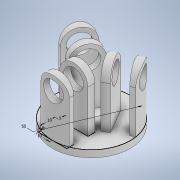
# Autodesk Inventor part: Base
Saved by Autodesk Inventor 2022 (Build 260153000, 153)
## iProperties
Created: 2022-10-13
Part Number: Base
Material: Generic
Document SubType Name: Modeling
Designer: Jasper
Density: 1 g/cm^3
Appearance: Default
Author: Jasper
Autodesk Inventor part; units mm, degrees
ref_plane "YZ Plane" through (0, 0, 0) normal (1, 0, 0) x (0, 1, 0)
ref_plane "XZ Plane" through (0, 0, 0) normal (0, 1, 0) x (-1, 0, 0)
ref_plane "XY Plane" through (0, 0, 0) normal (0, 0, 1) x (1, 0, 0)
sketch "Sketch1" plane through (0, 0, 0) normal (0, 1, 0) x (-1, 0, 0)
  circle A0 centre (0, 0) radius 27.5
  line L0 (0, 27.5) -> (10, 27.5)
  line L1 (10, 27.5) -> (10, 22.5)
  line L2 (10, 22.5) -> (0, 22.5)
  line L3 (0, 22.5) -> (0, 27.5)
  line L4 (10, 12.5) -> (0, 12.5)
  line L5 (0, 12.5) -> (0, 7.5)
  line L6 (0, 7.5) -> (10, 7.5)
  line L7 (10, 7.5) -> (10, 12.5)
  line L8 (0, 27.5) -> (-10, 27.5)
  line L9 (-10, 27.5) -> (-10, 22.5)
  line L10 (-10, 22.5) -> (0, 22.5)
  line L11 (-10, 12.5) -> (0, 12.5)
  line L12 (0, 7.5) -> (-10, 7.5)
  line L13 (-10, 7.5) -> (-10, 12.5)
  point P0 (-10, 25.6174)
  point P1 (10, 25.6174)
  dimension "d0" = 55
  dimension "d1" = 5
  dimension "d2" = 5
  dimension "d3" = 10
  dimension "d4" = 10
  constraints: 28 end point, 4 parallel, 4 symmetric about line, 3 point on line, 2 coincident, 2 horizontal, 2 perpendicular, 1 centre point, 1 tangent, 1 vertical alignment
  measures "d0" diameter of A0
  measures "d1" distance of L0.end L1.end
  measures "d2" distance of L6.end L4.start
  measures "d3" distance of L0.start L0.end
  measures "d4" distance between parallel lines of L4 L2
extrude "Extrusion1" add sketch "Sketch1" along normal blind 40 contours L1 L2 L3 A0 | A0 L3 L10 L9 | L7 L6 L5 L4 | L5 L12 L13 L11
extrude "Extrusion2" add sketch "Sketch1" against normal blind 5 contours A0 L9 L10 L2 L1 | L1 L2 L3 A0 | A0 L3 L10 L9 | L7 L6 L5 L4 | L5 L12 L13 L11
sketch "Sketch2" plane through (-10, 40, 12.5) normal (0, 0, 1) x (1, 0, 0)
  line L0 (20, -40) -> (20, 0) projected
  arc A0 (20, -10) -> (0.0697, -11.1785) centre (10, -10) ccw
  line L1 (0, 0) -> (20, 0) projected
  line L2 (0, -40) -> (0, 0) projected
  circle A1 centre (10, -10) radius 7
  point P0 (10, -40)
  point P1 (10, 0)
  point P2 (0, -10)
  dimension "d12" = 14
  constraints: 3 tangent, 2 centre point, 2 point on circle, 1 coincident, 1 point on line
  measures "d12" diameter of A1
extrude "Extrusion3" cut sketch "Sketch2" along normal blind 20 and the other way blind 5
pattern_circular "Circular Pattern1" count 3 over 360 about axis through (0, 0, 0) along (0, 1, 0) of "Extrusion1", "Extrusion2", "Extrusion3"
body "Solid1"
